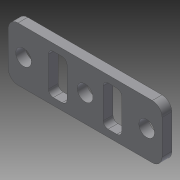
# Autodesk Inventor part: Vertical_Lead_Screw_E-stop_Plate
Saved by Autodesk Inventor 2015 (Build 190159000, 159)
## iProperties
Created: 2015-01-06
Part Number: Vertical_Lead_Screw_E-stop_Plate
Material: Generic
Document SubType Name: Modeling
Designer: Drew
Density: 1 g/cm^3
Appearance: Default
Author: Drew
Autodesk Inventor part; units mm, degrees
ref_plane "YZ Plane" through (0, 0, 0) normal (1, 0, 0) x (0, 1, 0)
ref_plane "XZ Plane" through (0, 0, 0) normal (0, 1, 0) x (-1, 0, 0)
ref_plane "XY Plane" through (0, 0, 0) normal (0, 0, 1) x (1, 0, 0)
sketch "Sketch1" plane through (0, 0, 0) normal (0, 0, 1) x (1, 0, 0)
  line L0 (43.65, -17.5) -> (-43.65, -17.5)
  line L1 (-50, -11.15) -> (-50, 11.15)
  line L2 (-43.65, 17.5) -> (43.65, 17.5)
  line L3 (50, 11.15) -> (50, -11.15)
  line L4 (50, -17.5) -> (-50, 17.5) construction
  line L5 (-50, -17.5) -> (50, 17.5) construction
  line L6 (0, 51.2558) -> (0, -45.9758)
  circle A0 centre (-40, 0) radius 5.1
  line L7 (-83.6339, 0) -> (65.0593, 0)
  circle A1 centre (40, 0) radius 5.1
  circle A2 centre (0, 0) radius 5.1
  arc A3 (-43.65, 17.5) -> (-50, 11.15) centre (-43.65, 11.15) ccw
  arc A4 (-50, -11.15) -> (-43.65, -17.5) centre (-43.65, -11.15) ccw
  arc A5 (43.65, -17.5) -> (50, -11.15) centre (43.65, -11.15) ccw
  arc A6 (50, 11.15) -> (43.65, 17.5) centre (43.65, 11.15) ccw
  line L8 (-14.905, -13) -> (-20.655, -13)
  line L9 (-23.83, -9.825) -> (-23.83, 9.825)
  line L10 (-20.655, 13) -> (-14.905, 13)
  line L11 (-11.73, 9.825) -> (-11.73, -9.825)
  line L12 (-11.73, -13) -> (-23.83, 13) construction
  line L13 (-23.83, -13) -> (-11.73, 13) construction
  line L14 (14.905, -13) -> (20.655, -13)
  line L15 (23.83, -9.825) -> (23.83, 9.825)
  line L16 (20.655, 13) -> (14.905, 13)
  line L17 (11.73, 9.825) -> (11.73, -9.825)
  line L18 (11.73, -13) -> (23.83, 13) construction
  line L19 (23.83, -13) -> (11.73, 13) construction
  arc A7 (-20.655, 13) -> (-23.83, 9.825) centre (-20.655, 9.825) ccw
  arc A8 (-11.73, 9.825) -> (-14.905, 13) centre (-14.905, 9.825) ccw
  arc A9 (-14.905, -13) -> (-11.73, -9.825) centre (-14.905, -9.825) ccw
  arc A10 (-23.83, -9.825) -> (-20.655, -13) centre (-20.655, -9.825) ccw
  arc A11 (11.73, -9.825) -> (14.905, -13) centre (14.905, -9.825) ccw
  arc A12 (20.655, -13) -> (23.83, -9.825) centre (20.655, -9.825) ccw
  arc A13 (23.83, 9.825) -> (20.655, 13) centre (20.655, 9.825) ccw
  arc A14 (14.905, 13) -> (11.73, 9.825) centre (14.905, 9.825) ccw
  point P0 (0, 0)
  point P1 (0, 0)
  point P2 (-17.78, 0)
  point P3 (17.78, 0)
  dimension "d0" = 100
  dimension "d1" = 35
  dimension "d2" = 80
  dimension "d3" = 10.2
  dimension "d6" = 10.2
  dimension "d7" = 6.35
  dimension "d8" = 26
  dimension "d9" = 12.1
  dimension "d10" = 3.175
  dimension "d11" = 35.56
  constraints: 40 end point, 28 point on line, 24 point on circle, 24 tangent, 15 centre point, 10 equal radius, 8 midpoint, 6 symmetric about line, 4 parallel, 3 horizontal, 2 perpendicular, 1 coincident, 1 vertical, 1 other
  measures "d0" distance of L4.end L5.end
  measures "d1" distance of L5.start L4.end
  measures "d2" diameter of A0.centre L6
  measures "d3" diameter of A0
  measures "d6" diameter of A2
  measures "d7" radius of A3
  measures "d8" distance of L13.start L12.end
  measures "d9" distance of L12.end L13.end
  measures "d10" radius of A7
  measures "d11" diameter of point (-17.78, 0) L6
extrude "Extrusion1" add sketch "Sketch1" along normal blind 6.35 contours L0 L6 A2 L7 L17 A11 L14 A12 L15 A1 L3 A5 | L0 A4 L1 L7 A0 L9 A10 L8 A9 L11 A2 L6 | L7 A1 L15 A13 L16 A14 L17 A2 L6 L2 A6 L3 | L7 L11 A8 L10 A7 L9 A0 L1 A3 L2 L6 A2
equation "\"d6\" = d3"
body "Solid1"
